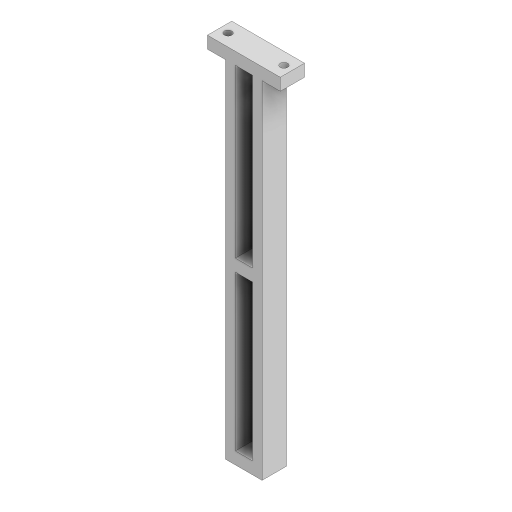
# Autodesk Inventor part: CenterSupport
Saved by Autodesk Inventor 2023 (Build 270158000, 158)
## iProperties
Created: 2023-10-19
Part Number: CenterSupport
Material: Generic
Document SubType Name: Modeling
Designer: MVeszpremi
Density: 1 g/cm^3
Appearance: Default
Author: MVeszpremi
Autodesk Inventor part; units mm, degrees
ref_plane "YZ Plane" through (0, 0, 0) normal (1, 0, 0) x (0, 1, 0)
ref_plane "XZ Plane" through (0, 0, 0) normal (0, 1, 0) x (-1, 0, 0)
ref_plane "XY Plane" through (0, 0, 0) normal (0, 0, 1) x (1, 0, 0)
sketch "Sketch1" plane through (0, 0, 0) normal (0, 0, 1) x (1, 0, 0)
  line L0 (-15, -0.0024) -> (15, -0.0024)
  line L1 (15, -0.0024) -> (15, 4.9976)
  line L2 (15, 4.9976) -> (-15, 4.9976)
  line L3 (-15, 4.9976) -> (-15, -0.0024)
  line L4 (-7.5, -0.0024) -> (7.5, -0.0024)
  line L5 (7.5, -0.0024) -> (7.5, -142.5024)
  line L6 (7.5, -142.5024) -> (-7.5, -142.5024)
  line L7 (-7.5, -142.5024) -> (-7.5, -0.0024)
  point P0 (0, 0)
  point P1 (0, -0.0024)
  point P2 (7.5, -0.0024)
  dimension "d0" = 5
  dimension "d1" = 147.5
  dimension "d3" = 7.5
  dimension "d5" = 30
  dimension "d6" = 15
  dimension "d7" = 7.5
  constraints: 16 end point, 4 parallel, 2 horizontal, 2 perpendicular, 1 midpoint, 1 point on line
  measures "d0" distance between parallel lines of L0 L2
  measures "d1" distance between parallel lines of L6 L2
  measures "d3" distance from line of L7 point (0, 0)
  measures "d5" distance of L1.end L2.end
  measures "d6" distance from line of point (0, 0) L1
  measures "d7" distance from line of point (0, -0.002) L5
extrude "Extrusion1" add sketch "Sketch1" along normal blind 10
sketch "Sketch2" plane through (0, 0, 10) normal (0, 0, 1) x (1, 0, 0)
  line L0 (-3.5, 0) -> (3.5, 0)
  line L1 (3.5, 0) -> (3.5, -137.5024)
  line L2 (3.5, -137.5024) -> (-3.5, -137.5024)
  line L3 (-3.5, -137.5024) -> (-3.5, 0)
  line L4 (-7.5, -0.0024) -> (-7.5, -142.5024) projected
  line L5 (7.5, -142.5024) -> (7.5, -0.0024) projected
  line L6 (-7.5, -142.5024) -> (7.5, -142.5024) projected
  line L7 (-3.5, -68.7512) -> (3.5, -68.7512)
  line L8 (3.5, -68.7512) -> (3.5, -73.7512)
  line L9 (3.5, -73.7512) -> (-3.5, -73.7512)
  line L10 (-3.5, -73.7512) -> (-3.5, -68.7512)
  point P0 (0, 0)
  point P1 (3.5, -68.7512)
  dimension "d10" = 4
  dimension "d11" = 4
  dimension "d12" = 5
  dimension "d13" = 5
  constraints: 16 end point, 4 parallel, 2 horizontal, 2 midpoint, 2 perpendicular, 1 point on line
  measures "d10" distance between parallel lines of L4 L3
  measures "d11" distance between parallel lines of L5 L1
  measures "d12" distance from line of L6 L1.end
  measures "d13" distance of L8.end point (3.5, -68.751)
extrude "Extrusion2" cut sketch "Sketch2" against normal blind 10 contours L0 L1 L7 L3 | L9 L1 L2 L3
sketch "Sketch3" plane through (7.5, -0.0024, 0) normal (0, -1, 0) x (1, 0, 0)
  circle A0 centre (4, 5) radius 1.5
  circle A1 centre (-19, 5) radius 1.5
  line L0 (7.5, 0) -> (7.5, 10) projected
  line L1 (0, 10) -> (7.5, 10) projected
  line L2 (-22.5, 10) -> (-15, 10) projected
  line L3 (-22.5, 0) -> (-22.5, 10) projected
  point P0 (-7.5, 0)
  point P1 (-18.75, 10)
  dimension "d16" = 3.5
  dimension "d17" = 5
  dimension "d19" = 5
  dimension "d20" = 3.5
  dimension "d21" = 3
  dimension "d22" = 3
  constraints: 2 centre point, 1 midpoint
  measures "d16" distance from line of L0 A0.centre
  measures "d17" distance from line of L1 A0.centre
  measures "d19" distance from line of L2 A1.centre
  measures "d20" distance from line of L3 A1.centre
  measures "d21" diameter of A1
  measures "d22" diameter of A0
extrude "Extrusion3" cut sketch "Sketch3" against normal blind 10
chamfer "Chamfer1" distance 1.5 angle 45 2 edges at (-13, -0.0024, 5) (10, -0.0024, 5)
body "Solid1"
